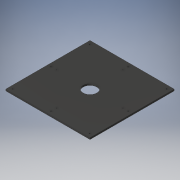
# Autodesk Inventor part: turntable-adapter-top
Saved by Autodesk Inventor 2019 (Build 230136000, 136)
## iProperties
Created: 2019-04-16
Part Number: turntable-adapter-top
Material: Acetal Resin, Black
Document SubType Name: Modeling
Designer: Wilson Lab
Density: 1.425 g/cm^3
Appearance: Smooth - Black
Author: Wilson Lab
Autodesk Inventor part; units mm, degrees
ref_plane "YZ Plane" through (0, 0, 0) normal (1, 0, 0) x (0, 1, 0)
ref_plane "XZ Plane" through (0, 0, 0) normal (0, 1, 0) x (-1, 0, 0)
ref_plane "XY Plane" through (0, 0, 0) normal (0, 0, 1) x (1, 0, 0)
sketch "Sketch1" plane through (0, 0, 0) normal (0, 1, 0) x (-1, 0, 0)
  line L0 (-152.4, 152.4) -> (152.4, 152.4)
  line L1 (152.4, 152.4) -> (152.4, -152.4)
  line L2 (152.4, -152.4) -> (-152.4, -152.4)
  line L3 (-152.4, -152.4) -> (-152.4, 152.4)
  line L4 (-152.4, 152.4) -> (152.4, -152.4) construction
  line L5 (152.4, 152.4) -> (-152.4, -152.4) construction
  point P0 (0, 0)
  dimension "d0" = 304.8
  constraints: 12 end point, 2 midpoint, 2 parallel, 2 perpendicular, 1 horizontal
  measures "d0" distance of L0.end L1.end
extrude "Extrusion1" add sketch "Sketch1" along normal blind 6.35
sketch "Sketch4" plane through (0, 6.35, 0) normal (0, 1, 0) x (1, 0, 0)
  line L0 (-152.4, -152.4) -> (152.4, -152.4) construction
  line L1 (152.4, -152.4) -> (152.4, 152.4) construction
  line L2 (152.4, 152.4) -> (-152.4, 152.4) construction
  line L3 (-152.4, 152.4) -> (-152.4, -152.4) construction
  line L4 (139.7, -139.7) -> (-139.7, -139.7) construction
  line L5 (-139.7, -139.7) -> (-139.7, 139.7) construction
  line L6 (-139.7, 139.7) -> (139.7, 139.7) construction
  line L7 (139.7, 139.7) -> (139.7, -139.7) construction
  line L8 (139.7, -139.7) -> (-139.7, 139.7) construction
  line L9 (-139.7, -139.7) -> (139.7, 139.7) construction
  point P0 (0, 0)
  point P1 (0, -139.7)
  point P2 (-139.7, 0)
  point P3 (0, 139.7)
  point P4 (139.7, 0)
  dimension "d21" = 279.4
  dimension "d22" = 279.4
  constraints: 12 end point, 6 midpoint, 4 coincident, 2 parallel, 1 horizontal, 1 perpendicular
  measures "d21" distance of L4.end L5.end
  measures "d22" distance between parallel lines of L7 L5
hole "Hole2" at (-139.7, 6.35, 139.7) at (0, 6.35, 139.7) at (-139.7, 6.35, 0) at (-139.7, 6.35, -139.7) at (0, 6.35, -139.7) at (139.7, 6.35, -139.7) at (139.7, 6.35, 0) at (139.7, 6.35, 139.7) direction (0, -1, 0) diameter 6.528 depth 19.05 tip angle 118 clearance for "Socket Head Cap Screw" size "1/4" standard "Ansi Unified Screw Threads"
sketch "Sketch2" plane through (0, 6.35, 0) normal (0, 1, 0) x (1, 0, 0)
  line L0 (-152.4, -152.4) -> (152.4, -152.4) construction
  line L1 (152.4, -152.4) -> (152.4, 152.4) construction
  line L2 (152.4, 152.4) -> (-152.4, 152.4) construction
  line L3 (-152.4, 152.4) -> (-152.4, -152.4) construction
  circle A0 centre (0, 0) radius 120.2565 construction
  line L4 (0, -152.4) -> (0, 152.4) construction
  line L5 (152.4, 152.4) -> (-152.4, 152.4) construction
  line L6 (-152.4, 0) -> (152.4, 0) construction
  point P0 (-120.2565, 0)
  point P1 (0, 120.2565)
  point P2 (120.2565, 0)
  point P3 (0, -120.2565)
  dimension "d3" = 240.513
  constraints: 4 end point, 4 midpoint, 4 point on circle, 4 point on line, 1 centre point, 1 coincident
  measures "d3" diameter of A0
hole "Hole1" at (-120.2565, 6.35, 0) at (0, 6.35, 120.2565) at (120.2565, 6.35, 0) at (0, 6.35, -120.2565) direction (0, -1, 0) diameter 4.978 depth 19.05 tip angle 118 thread size "1/4-20 UNC" class "2B" standard "ANSI Unified Screw Threads"
sketch "Sketch3" plane through (0, 6.35, 0) normal (0, 1, 0) x (1, 0, 0)
  line L0 (-152.4, -152.4) -> (152.4, -152.4) projected
  line L1 (152.4, -152.4) -> (152.4, 152.4) projected
  line L2 (152.4, 152.4) -> (-152.4, 152.4) projected
  line L3 (-152.4, 152.4) -> (-152.4, -152.4) projected
  circle A0 centre (0, 0) radius 25
  dimension "d18" = 50
  constraints: 1 centre point, 1 coincident
  measures "d18" diameter of A0
extrude "Extrusion3" cut sketch "Sketch3" against normal through all contours A0
body "Solid1"
